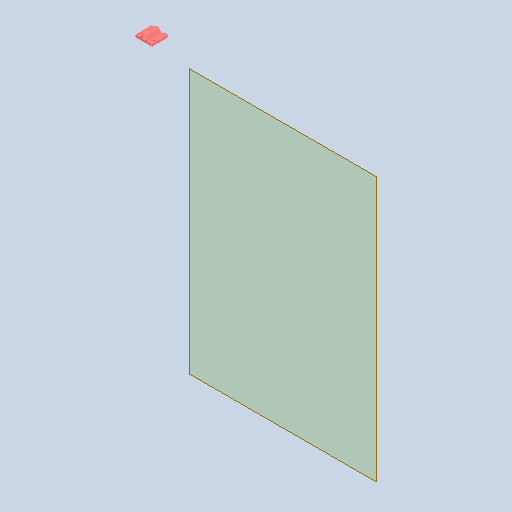
# Autodesk Inventor part: AxleHolder
Saved by Autodesk Inventor 2023 (Build 270158000, 158)
## iProperties
Created: 2023-08-18
Part Number: AxleHolder
Material: Generic
Document SubType Name: Modeling
Designer: Felix
Density: 1 g/cm^3
Appearance: Smooth - Red
Author: Felix
Autodesk Inventor part; units mm, degrees
ref_plane "YZ Plane" through (0, 0, 0) normal (1, 0, 0) x (0, 1, 0)
ref_plane "XZ Plane" through (0, 0, 0) normal (0, 1, 0) x (-1, 0, 0)
ref_plane "XY Plane" through (0, 0, 0) normal (0, 0, 1) x (1, 0, 0)
ref_plane "Work Plane2" through (234.4934, -62.0868, 206.5159) normal (0, 0, -1) x (-1, 0, 0)
sketch "Sketch3" plane through (234.4934, -62.0868, 206.5159) normal (0, 0, -1) x (-1, 0, 0)
  circle A0 centre (304.3, 375) radius 4 construction
  line L0 (294.485, 372) -> (300.2585, 382)
  line L1 (300.2585, 382) -> (308.3415, 382)
  line L2 (308.3415, 382) -> (314.115, 372)
  line L3 (-365, 367) -> (365, 367) construction
  line L4 (294.485, 372) -> (294.485, 367) construction
  line L5 (314.115, 372) -> (314.115, 367) construction
  line L6 (294.485, 372) -> (284.485, 372)
  line L7 (284.485, 372) -> (284.485, 367)
  line L8 (284.485, 367) -> (294.485, 367)
  line L9 (294.485, 367) -> (294.485, 372) construction
  line L10 (314.115, 372) -> (324.115, 372)
  line L11 (324.115, 372) -> (324.115, 367)
  line L12 (324.115, 367) -> (314.115, 367)
  line L13 (314.115, 367) -> (314.115, 372) construction
  line L14 (294.485, 367) -> (314.115, 367)
  point P0 (234.4934, 62.0868)
  dimension "d19" = 8
  dimension "d20" = 3
  dimension "d21" = 60
  dimension "d22" = 60
  dimension "d24" = 3
  dimension "d25" = 3
  dimension "d26" = 5
  dimension "d27" = 5
  dimension "d28" = 10
  dimension "d29" = 10
  constraints: 28 end point, 4 parallel, 4 perpendicular, 4 point on line, 3 horizontal, 1 centre point, 1 coincident, 1 collinear
  measures "d19" diameter of A0
  measures "d20" distance edge to line of A0 L1
  measures "d21" angle of L1 L0
  measures "d22" angle of L1 L2
  measures "d24" distance edge to line of A0 L0
  measures "d25" distance edge to line of A0 L2
  measures "d26" distance of L0.start L4.end
  measures "d27" distance of L2.end L5.end
  measures "d28" distance of L0.start L6.end
  measures "d29" distance of L2.end L10.end
ref_plane "Work Plane3" through (-75.5066, 299.1132, 245.5159) normal (0, 0, 1) x (1, 0, 0)
extrude "Extrusion2" add sketch "Sketch3" against normal up to surface (39 mm away)
sketch "Sketch4" plane through (234.4934, -62.0868, 206.5159) normal (0, 0, -1) x (-1, 0, 0)
  point P0 (234.4934, 62.0868)
  point P1 (304.3, 375)
hole "Hole2" at (-69.8066, 312.9132, 206.5159) direction (0, 0, 1) diameter 8.4 end through all counterbore diameter 18 counterbore depth 6.3 clearance for "Hex Head Cap Screw DIN EN 24017" size "M8" standard "DIN"
sketch "Sketch5" plane through (-59.9916, 309.9132, 206.5159) normal (0, 1, 0) x (1, 0, 0)
  line L0 (-139.515, -29) -> (728.485, -29) construction
  line L1 (-139.515, -9) -> (728.485, -9) construction
  line L2 (10, 0) -> (10, -39) construction
  line L3 (-29.6299, 0) -> (-29.6299, -39) construction
  point P0 (59.9916, 206.5159)
  point P1 (5, -29)
  point P2 (-24.6299, -29)
  point P3 (-24.6299, -9)
  point P4 (5, -9)
  dimension "d39" = 5
  dimension "d40" = 5
  dimension "d41" = 5
  dimension "d42" = 5
  constraints: 4 point on line
  measures "d39" distance from line of L2 point (5, -29)
  measures "d40" distance from line of L3 point (-24.63, -29)
  measures "d41" distance from line of L2 point (5, -9)
  measures "d42" distance from line of L3 point (-24.63, -9)
hole "Hole3" at (-54.9916, 309.9132, 235.5159) at (-84.6215, 309.9132, 235.5159) at (-84.6215, 309.9132, 215.5159) at (-54.9916, 309.9132, 215.5159) direction (0, -1, 0) diameter 5.3 end through all clearance for "Hex Head Cap Screw DIN EN 24017" size "M5" standard "DIN"
sketch "Sketch6" plane through (-59.9916, 309.9132, 206.5159) normal (0, 1, 0) x (1, 0, 0)
  point P0 (59.9916, 206.5159)
  point P1 (5, -29)
  point P2 (-24.6299, -29)
  point P3 (-24.6299, -9)
  point P4 (5, -9)
hole "Hole4" at (-54.9916, 309.9132, 235.5159) at (-84.6215, 309.9132, 235.5159) at (-84.6215, 309.9132, 215.5159) at (-54.9916, 309.9132, 215.5159) direction (0, 1, 0) diameter 11 end through all
sketch "Sketch7" plane through (234.4934, -62.0868, 206.5159) normal (0, 0, -1) x (-1, 0, 0)
  arc A0 (295.4094, 373.601) -> (300.1769, 367) centre (304.3, 375) ccw projected
  line L0 (295.4094, 373.601) -> (294.485, 372) projected
  line L1 (294.485, 372) -> (284.485, 372) projected
  line L2 (284.485, 372) -> (284.485, 367) projected
  line L3 (284.485, 367) -> (300.1769, 367) projected
  arc A1 (308.4231, 367) -> (313.1906, 373.601) centre (304.3, 375) ccw projected
  line L4 (308.4231, 367) -> (324.115, 367) projected
  line L5 (324.115, 367) -> (324.115, 372) projected
  line L6 (324.115, 372) -> (314.115, 372) projected
  line L7 (314.115, 372) -> (313.1906, 373.601) projected
  line L8 (294.485, 372) -> (297.3718, 367)
  line L9 (314.115, 372) -> (311.2282, 367)
  line L10 (284.485, 367) -> (324.115, 367) projected
  point P0 (234.4934, 62.0868)
  dimension "d59" = 60
  dimension "d60" = 60
  constraints: 4 end point, 2 point on line
  measures "d59" angle of L1 L8
  measures "d60" angle of L6 L9
extrude "Extrusion3" cut sketch "Sketch7" against normal up to surface (6.3 mm away) contours A0 L3 L8 L0 | A1 L7 L9 L4
equation "\"d22\" = d21"
equation "\"d24\" = d20"
equation "\"d25\" = d24"
equation "\"d27\" = d26"
equation "\"d29\" = d28"
equation "\"d40\" = d39"
equation "\"d41\" = d39"
equation "\"d42\" = d39"
equation "\"d60\" = d59"
body "Solid2"
